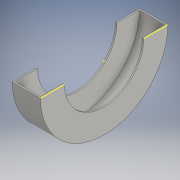
# Autodesk Inventor part: Holster
Saved by Autodesk Inventor 2016 (Build 200138000, 138)
## iProperties
Created: 2017-01-08
Part Number: Holster
Material: Generic
Document SubType Name: Modeling
Designer: madsenn
Density: 1 g/cm^3
Appearance: Default
Author: madsenn
Autodesk Inventor part; units mm, degrees
ref_plane "YZ Plane" through (0, 0, 0) normal (1, 0, 0) x (0, 1, 0)
ref_plane "XZ Plane" through (0, 0, 0) normal (0, 1, 0) x (-1, 0, 0)
ref_plane "XY Plane" through (0, 0, 0) normal (0, 0, 1) x (1, 0, 0)
sketch "Sketch1" plane through (0, 0, 0) normal (0, 1, 0) x (-1, 0, 0)
  arc A0 (139.7, 0) -> (-139.7, 0) centre (0, 0) ccw
  arc A1 (142.875, 0) -> (-142.875, 0) centre (0, 0) ccw
  line L0 (139.7, 0) -> (142.875, 0)
  line L1 (-139.7, 0) -> (-142.875, 0)
  dimension "d0" = 279.4
  dimension "d1" = 3.175
  constraints: 4 end point, 4 point on circle, 2 centre point, 2 coincident, 1 point on line
  measures "d0" diameter of A0
  measures "d1" radial gap between concentric circles of A1 A0
extrude "Extrusion1" add sketch "Sketch1" along normal blind 57.15
sketch "Sketch2" plane through (0, 57.15, 0) normal (0, 1, 0) x (1, 0, 0)
  arc A0 (-88.9, 0) -> (88.9, 0) centre (0, 0) ccw
  arc A1 (-142.875, 0) -> (142.875, 0) centre (0, 0) ccw projected
  line L0 (-139.7, 0) -> (-142.875, 0) projected
  line L1 (-142.875, 0) -> (-88.9, 0)
  line L2 (88.9, 0) -> (142.875, 0)
  dimension "d4" = 177.8
  constraints: 4 end point, 2 collinear, 2 point on circle, 1 centre point, 1 coincident
  measures "d4" diameter of A0
extrude "Extrusion2" add sketch "Sketch2" along normal blind 3.175
sketch "Sketch3" plane through (0, 0, 0) normal (0, -1, 0) x (1, 0, 0)
  arc A0 (142.875, 0) -> (-142.875, 0) centre (0, 0) ccw projected
  arc A1 (88.9, 0) -> (-88.9, 0) centre (0, 0) ccw projected
  line L0 (-139.7, 0) -> (-88.9, 0) projected
  line L1 (88.9, 0) -> (139.7, 0) projected
  line L2 (139.7, 0) -> (142.875, 0) projected
  line L3 (-142.875, 0) -> (-139.7, 0) projected
extrude "Extrusion3" add sketch "Sketch3" along normal blind 3.175
sketch "Sketch4" plane through (0, 60.325, 0) normal (0, 1, 0) x (1, 0, 0)
  line L0 (-88.9, 0) -> (-142.875, 0) projected
  line L1 (142.875, 0) -> (88.9, 0) projected
  point P0 (0, 0)
body "Solid1"
